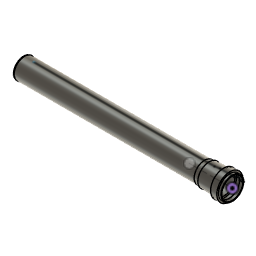
KG ROhr DN50x500 v2 (Autodesk Fusion 360 design; units mm, degrees)
Autodesk Fusion 360 part; units mm, degrees
sketch "Skizze1" plane through (0, 0, 0) normal (0, 0, 1) x (1, 0, 0)
  line L0 (-502.8868, 23) -> (-66.7976, 23)
  line L1 (-66.7976, 23) -> (-55.7976, 25.25)
  line L2 (-55.7976, 25.25) -> (-19, 25.25)
  line L3 (-19, 25.25) -> (-19, 29.5)
  line L4 (-19, 29.5) -> (-8, 29.5)
  line L5 (-8, 29.5) -> (-8, 25.5)
  line L6 (-8, 25.5) -> (0, 25.5)
  line L7 (0, 27.5) -> (-6, 27.5)
  line L8 (-6, 27.5) -> (-6, 31.5)
  line L9 (-6, 31.5) -> (-21, 31.5)
  line L10 (-21, 31.5) -> (-21, 27.25)
  line L11 (-21, 27.25) -> (-56, 27.25)
  line L12 (-56, 27.25) -> (-67, 25)
  line L13 (-67, 25) -> (-500.8868, 25)
  line L14 (0, 0) -> (-103.5201, 0)
  line L15 (-502.8868, 23) -> (-502.8868, 24.4641)
  line L16 (-502.8868, 24.4641) -> (-500.8868, 25)
  line L17 (0, 25.5) -> (0, 27.5)
  dimension "d2" = 15
  dimension "d3" = 2
  dimension "d4" = 2
  dimension "d5" = 63
  dimension "d6" = 2
  dimension "d7" = 55
  dimension "d8" = 54.5
  dimension "d10" = 50
  dimension "d12" = 2
  dimension "d13" = 2
  dimension "d14" = 2
  dimension "d15" = 35
  dimension "d16" = 46
  dimension "d17" = 2
  dimension "d18" = 2
  dimension "d19" = 15
  dimension "d21" = 6
  constraint horizontal L0
  constraint parallel L0 L2
  constraint perpendicular L2 L3
  constraint perpendicular L3 L4
  constraint perpendicular L4 L5
  constraint perpendicular L5 L6
  constraint perpendicular L7 L8
  constraint perpendicular L8 L9
  constraint perpendicular L9 L10
  constraint perpendicular L10 L11
  constraint coincident L14.start origin
  constraint parallel L11 L14
  constraint horizontal L13
  constraint parallel L1 L12
  constraint perpendicular L0 L15
  constraint perpendicular L7 L17
  constraint coincident L14.start L17
  measures "d2" distance of L8.end L9.end
  measures "d3" distance of L3 L10
  measures "d4" distance of L5 L8
  measures "d6" distance of L4 L9
  measures "d12" distance of L2 L11
  measures "d13" distance of L1 L12
  measures "d14" distance of L6 L7
  measures "d15" distance of L10.end L11.end
  measures "d16" distance of L10 L12.end
  measures "d17" distance of L0 L13
  measures "d18" distance of L13.end L15
  measures "d19" angle of L13 L16
  measures "d21" distance of L8 L17
revolve "Drehen1" add sketch "Skizze1" angle 360 about axis through (0, 0, 0) along (-1, 0, 0)
